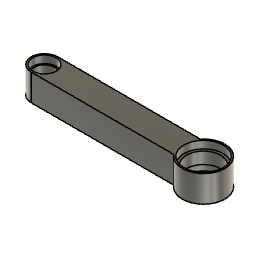
Distal arm v1 (Autodesk Fusion 360 design; units mm, degrees)
Autodesk Fusion 360 part; units mm, degrees
note: some values were not read from the file. Set by a fixed rule: which sketch regions a step uses.
sketch "Sketch1" plane through (0, 0, 0) normal (0, 0, 1) x (1, 0, 0)
  circle A0 centre (0, 0) radius 12.5
  line L0 (0, -12.5) -> (150, -12.5)
  line L1 (150, -12.5) -> (150, 12.5)
  line L2 (150, 12.5) -> (0, 12.5)
  line L3 (0, 12.5) -> (0, -12.5)
  circle A1 centre (150, 0) radius 20
  dimension "d1" = 25
  dimension "d2" = 25
  dimension "d3" = 150
  constraint coincident A0.centre origin
  constraint horizontal L0
  constraint vertical L1
  constraint horizontal L2
  constraint vertical L3
  constraint coincident A0 L0.start
  constraint midpoint L1 A1.centre
  measures "d1" diameter of A0
  measures "d2" distance of L0.start L2.end
  measures "d3" distance of L0.start L0.end
extrude "Extrude1" add sketch "Sketch1" along normal blind 25 makes body 1
sketch "Sketch2" plane through (0, 0, 0) normal (0, 0, 1) x (1, 0, 0)
  circle A0 centre (150, 0) radius 18.5
  dimension "d6" = 37
  measures "d6" diameter of A0
extrude "Extrude2" cut sketch "Sketch2" along normal mid plane 7 bodies 1
sketch "Sketch3" plane through (0, 0, 25) normal (0, 0, 1) x (-1, 0, 0)
  arc A0 (-134.3875, 12.5) -> (-134.3875, -12.5) centre (-150, 0) ccw
  line L0 (-134.3875, -12.5) -> (0, -12.5)
  arc A1 (0, -12.5) -> (0, 12.5) centre (0, 0) ccw
  line L1 (0, 12.5) -> (-134.3875, 12.5)
  circle A2 centre (-150, 0) radius 18.5
  dimension "d9" = 37
  constraint concentric A0 A2
  measures "d9" diameter of A2
extrude "Extrude3" cut sketch "Sketch3" against normal blind 7 contours A2 bodies 1
sketch "Sketch4" plane through (0, 0, 3.5) normal (0, 0, -1) x (1, 0, 0)
  circle A0 centre (150, 0) radius 18.5
extrude "Extrude4" cut sketch "Sketch4" against normal blind 3.5 bodies 1
sketch "Sketch5" plane through (0, 0, 18) normal (0, 0, 1) x (-1, 0, 0)
  circle A0 centre (-150, 0) radius 18.5
  circle A1 centre (-150, 0) radius 12.5
  dimension "d14" = 25
  constraint concentric A0 A1
  measures "d14" diameter of A1
extrude "Extrude5" cut sketch "Sketch5" against normal through all contours A1 bodies 1
sketch "Sketch6" plane through (0, 0, 0) normal (0, 0, 1) x (1, 0, 0)
  circle A0 centre (0, 0) radius 11
  dimension "d16" = 22
  constraint coincident A0.centre origin
  measures "d16" diameter of A0
extrude "Extrude6" cut sketch "Sketch6" along normal blind 7 bodies 1
sketch "Sketch7" plane through (0, 0, 25) normal (0, 0, 1) x (-1, 0, 0)
  circle A0 centre (-150, 0) radius 18.5
  arc A1 (-134.3875, 12.5) -> (-134.3875, -12.5) centre (-150, 0) ccw
  line L0 (-134.3875, -12.5) -> (0, -12.5)
  arc A2 (0, -12.5) -> (0, 12.5) centre (0, 0) ccw
  line L1 (0, 12.5) -> (-134.3875, 12.5)
  circle A3 centre (0, 0) radius 11
  dimension "d19" = 22
  constraint coincident A2.centre A3.centre
  measures "d19" diameter of A3
extrude "Extrude7" cut sketch "Sketch7" against normal blind 7 contours A3 bodies 1
sketch "Sketch8" plane through (0, 0, 25) normal (0, 0, 1) x (-1, 0, 0)
  circle A0 centre (0, 0) radius 11
  circle A1 centre (-150, 0) radius 18.5
  arc A2 (-134.3875, 12.5) -> (-134.3875, -12.5) centre (-150, 0) ccw
  line L0 (-134.3875, -12.5) -> (0, -12.5)
  arc A3 (0, -12.5) -> (0, 12.5) centre (0, 0) ccw
  line L1 (0, 12.5) -> (-134.3875, 12.5)
  circle A4 centre (0, 0) radius 9.5
  dimension "d22" = 19
  constraint coincident A0.centre A3.centre
  measures "d22" diameter of A4
extrude "Extrude8" cut sketch "Sketch8" against normal through all contours A4 bodies 1
sketch "Sketch9" plane through (0, 0, 0) normal (0, 0, 1) x (1, 0, 0)
  circle A0 centre (150, 0) radius 16
  dimension "d25" = 32
  measures "d25" diameter of A0
extrude "Extrude9" cut sketch "Sketch9" along normal through all bodies 1
copy_body "Body->Comp1" bodies 1 removing the originals makes body 2 in component "Component"
copy_body "CopyPasteBodies1" bodies 2 makes body 3 in component "Component"
move_body "Move1" bodies 3 to x (1, 0, 0) y (0, 1, 0) z (0, 0, 1) at (-73.4204, 59.4482, -30.963) in component "Component"
move_body "Move2" bodies 3 to x (1, 0, 0) y (0, 1, 0) z (0, 0, 1) at (-71.2674, -18.2917, 54.7249) in component "Component"
sketch "Sketch1 (2)" plane through (0, 0, 0) normal (0, 0, 1) x (1, 0, 0) in component "Component"
sketch "Sketch2 (2)" plane through (0, 0, 0) normal (0, 0, 1) x (1, 0, 0) in component "Component"
sketch "Sketch3 (2)" plane through (0, 0, 0) normal (0, 0, 1) x (1, 0, 0) in component "Component"
component "Component" placed x (1, 0, 0) y (0, 1, 0) z (0, 0, 1) at (-125.0256, 77.3225, 0)
hidden bodies 2
equation "d16 = 25 mm - 3 mm"
